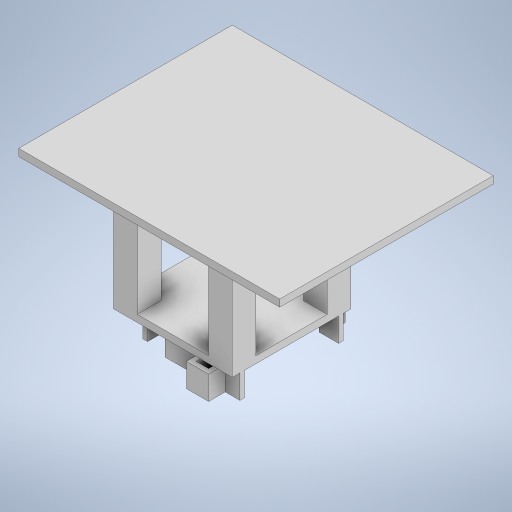
# Autodesk Inventor part: pitchrollmount44
Saved by Autodesk Inventor 2024 (Build 280153020, 153B)
## iProperties
Created: 2024-03-15
Part Number: pitchrollmount44
Material: Generic
Document SubType Name: Modeling
Designer: josep
Density: 1 g/cm^3
Appearance: Default
Author: josep
Autodesk Inventor part; units mm, degrees
ref_plane "YZ Plane" through (0, 0, 0) normal (1, 0, 0) x (0, 1, 0)
ref_plane "XZ Plane" through (0, 0, 0) normal (0, 1, 0) x (-1, 0, 0)
ref_plane "XY Plane" through (0, 0, 0) normal (0, 0, 1) x (1, 0, 0)
sketch "Sketch1" plane through (0, 0, 0) normal (0, 1, 0) x (-1, 0, 0)
  line L0 (25, 25) -> (15, 25)
  line L1 (15, 25) -> (15, 15)
  line L2 (15, 15) -> (25, 15)
  line L3 (25, 15) -> (25, 25)
  line L4 (25, 25) -> (-25, 25)
  line L5 (-25, 25) -> (-25, -25)
  line L6 (-25, -25) -> (25, -25)
  line L7 (25, -25) -> (25, 25)
  line L8 (25, 0) -> (-25, 0)
  line L9 (0, 25) -> (0, -25)
  line L10 (-25, 25) -> (-25, 15)
  line L11 (-15, 25) -> (-25, 25)
  line L12 (-15, 15) -> (-15, 25)
  line L13 (-25, 15) -> (-15, 15)
  line L14 (15, -15) -> (15, -25)
  line L15 (25, -15) -> (15, -15)
  line L16 (25, -25) -> (25, -15)
  line L17 (15, -25) -> (25, -25)
  line L18 (-25, -15) -> (-25, -25)
  line L19 (-15, -15) -> (-25, -15)
  line L20 (-15, -25) -> (-15, -15)
  line L21 (-25, -25) -> (-15, -25)
  line L22 (45, 45) -> (-45, 45)
  line L23 (-45, 45) -> (-45, -45)
  line L24 (-45, -45) -> (45, -45)
  line L25 (45, -45) -> (45, 45)
  point P0 (0, 0)
  point P1 (20, 25)
  point P2 (-20, 25)
  point P3 (20, -15)
  point P4 (-20, -15)
  point P5 (0, 45)
  dimension "d0" = 10
  dimension "d1" = 10
  dimension "d2" = 0
  dimension "d3" = 0
  dimension "d4" = 0
  dimension "d5" = 0
  dimension "d8" = 40
  dimension "d11" = 40
  dimension "d14" = 50
  dimension "d15" = 50
  dimension "d42" = 20
  dimension "d43" = 20
  dimension "d44" = 20
  dimension "d45" = 20
  constraints: 52 end point, 6 midpoint, 6 parallel, 4 horizontal, 4 perpendicular, 1 vertical, 27 other
  measures "d0" distance of L2.end L0.start
  measures "d1" distance between parallel lines of L3 L1
  measures "d2" vertical distance of L8.start point (0, 0)
  measures "d3" horizontal distance of L9.end point (0, 0)
  measures "d4" distance between parallel lines of L7 L3
  measures "d5" distance from line of L4 point (20, 25)
  measures "d8" distance of L0.end L10.start
  measures "d11" distance of L0.end L14.start
  measures "d14" distance of L6.end L4.start
  measures "d15" distance of L5.end L6.end
  measures "d42" distance between parallel lines of L25 L7
  measures "d43" distance from line of point (0, 45) L4
  measures "d44" distance between parallel lines of L24 L6
  measures "d45" distance between parallel lines of L23 L5
extrude "Extrusion1" add sketch "Sketch1" along normal blind 3 contours L1 L2 L7 L8 L9 L4 | L9 L8 L5 L13 L12 L4 | L7 L15 L14 L6 L9 L8 | L9 L6 L20 L19 L5 L8
extrude "Extrusion2" add sketch "Sketch1" along normal blind 55.594 contours L3 L2 L1 L0 | L12 L13 L5 L4 | L7 L6 L14 L15 | L19 L20 L6 L5
sketch "Sketch2" plane through (0, 0, 0) normal (0, -1, 0) x (1, 0, 0)
  line L0 (25, 15) -> (25, -15) projected
  line L1 (25, -19.8) -> (-15.893, -19.8)
  line L2 (-15.893, -19.8) -> (-15.893, 19.8)
  line L3 (-15.893, 19.8) -> (25, 19.8)
  line L4 (25, 19.8) -> (25, -19.8)
  line L5 (16.82, -19.8) -> (11.514, -19.8)
  line L6 (11.514, -19.8) -> (11.514, -26.8)
  line L7 (11.514, -26.8) -> (16.82, -26.8)
  line L8 (16.82, -26.8) -> (16.82, -19.8)
  line L9 (-15.893, 0) -> (25, 0)
  line L10 (11.514, 19.8) -> (11.514, 26.8)
  line L11 (11.514, 26.8) -> (16.82, 26.8)
  line L12 (16.82, 26.8) -> (16.82, 19.8)
  line L13 (-9.486, 19.8) -> (-5.486, 19.8)
  line L14 (9.514, 21.8) -> (-6.486, 21.8)
  line L15 (9.514, 21.8) -> (9.514, 28.8)
  line L16 (9.514, 28.8) -> (18.82, 28.8)
  line L17 (18.82, 28.8) -> (18.82, 21.8)
  line L18 (18.82, 21.8) -> (25, 21.8)
  line L19 (25, -15) -> (25, -25) projected
  line L20 (25, -21.8) -> (18.82, -21.8)
  line L21 (18.82, -21.8) -> (18.82, -28.8)
  line L22 (18.82, -28.8) -> (9.514, -28.8)
  line L23 (9.514, -28.8) -> (9.514, -21.8)
  line L24 (9.514, -21.8) -> (1.695, -21.8)
  line L25 (1.695, -21.8) -> (-17.893, -21.8)
  line L26 (-17.893, -21.8) -> (-17.893, 21.8)
  line L27 (25, 19.8) -> (25, 21.8)
  line L28 (25, -15) -> (25, -19.8)
  line L29 (25, -21.8) -> (25, -15)
  line L30 (-15.893, 19.8) -> (-17.893, 19.8)
  line L31 (-6.486, 21.8) -> (-6.486, 19.8)
  point P0 (0, 0)
  point P1 (16.82, -23.3)
  point P2 (4.5535, -19.8)
  point P3 (18.82, -25.3)
  point P4 (14.167, 28.8)
  point P5 (14.167, 26.8)
  point P6 (11.514, 23.3)
  point P7 (16.82, 19.8)
  point P8 (25, 14.5)
  point P9 (11.514, 19.8)
  point P10 (11.514, -19.8)
  point P11 (14.167, -28.8)
  dimension "d20" = 39.6
  dimension "d22" = 40.893
  dimension "d23" = 8.18
  dimension "d25" = 5.306
  dimension "d26" = 7
  dimension "d30" = 2
  dimension "d31" = 2
  dimension "d32" = 2
  dimension "d33" = 2
  dimension "d36" = 2
  dimension "d37" = 2
  dimension "d38" = 2
  dimension "d53" = 0
  dimension "d54" = 16
  dimension "d55" = 2
  dimension "d56" = 2
  constraints: 60 end point, 12 point on line, 9 midpoint, 9 perpendicular, 5 horizontal, 4 parallel, 4 symmetric about line, 2 collinear, 2 vertical
  measures "d20" distance of L1.end L2.end
  measures "d22" distance of L2.end L3.end
  measures "d23" distance from line of point (16.82, -23.3) L0
  measures "d25" distance of L6.end L7.end
  measures "d26" distance of L6.end L5.end
  measures "d30" distance between parallel lines of L1 L20
  measures "d31" distance from line of point (18.82, -25.3) L8
  measures "d32" distance between parallel lines of L6 L23
  measures "d33" distance between parallel lines of L2 L26
  measures "d36" distance between parallel lines of L14 L3
  measures "d37" distance of point (14.167, 28.8) point (14.167, 26.8)
  measures "d38" distance from line of L15 point (11.514, 23.3)
  measures "d53" vertical distance of point (0, 0) L9.end
  measures "d54" distance from line of L14.end L15
  measures "d55" distance from line of point (14.167, -28.8) L7
  measures "d56" distance between parallel lines of L12 L17
extrude "Extrusion3" add sketch "Sketch2" along normal blind 10 contours L3 L12 L11 L10 L31 L14 L15 L16 L17 L18 L27 | L2 L1 L6 L7 L8 L19 L20 L21 L22 L23 L24 L25 L26 L30
sketch "Sketch3" plane through (0, 55.594, 0) normal (0, 1, 0) x (1, 0, 0)
  line L0 (-45, -45) -> (65, -45)
  line L1 (65, -45) -> (65, 45)
  line L2 (65, 45) -> (-45, 45)
  line L3 (-45, 45) -> (-45, -45)
  line L4 (-25, -25) -> (-15, -25) projected
  line L5 (25, -25) -> (25, -15) projected
  line L6 (15, 25) -> (-15, 25) projected
  line L7 (-25, 15) -> (-25, -15) projected
  point P0 (0, 0)
  dimension "d46" = 20
  dimension "d47" = 40
  dimension "d48" = 20
  dimension "d49" = 20
  constraints: 8 end point, 2 parallel, 1 horizontal, 1 perpendicular
  measures "d46" distance between parallel lines of L4 L0
  measures "d47" distance between parallel lines of L5 L1
  measures "d48" distance between parallel lines of L2 L6
  measures "d49" distance between parallel lines of L7 L3
extrude "Extrusion4" add sketch "Sketch3" along normal blind 3
body "Solid1"
